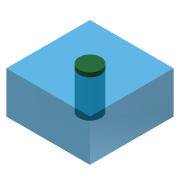
# Autodesk Inventor part: Remnant
Saved by Autodesk Inventor 2014 (Build 180170000, 170)
## iProperties
Created: 2015-06-22
Part Number: Remnant
Material: Generic
Document SubType Name: Modeling
Designer: kulkarni
Density: 1 g/cm^3
Appearance: Default
Author: kulkarni
Autodesk Inventor part; units mm, degrees
ref_plane "YZ Plane" through (0, 0, 0) normal (1, 0, 0) x (0, 1, 0)
ref_plane "XZ Plane" through (0, 0, 0) normal (0, 1, 0) x (-1, 0, 0)
ref_plane "XY Plane" through (0, 0, 0) normal (0, 0, 1) x (1, 0, 0)
sketch "Sketch1" plane through (0, 0, 0) normal (0, 1, 0) x (-1, 0, 0)
  line L0 (0, 0) -> (25.4, 0)
  line L1 (25.4, 0) -> (25.4, -25.4)
  line L2 (25.4, -25.4) -> (0, -25.4)
  line L3 (0, -25.4) -> (0, 0)
  dimension "d0" = 25.4
  dimension "d1" = 25.4
  constraints: 8 end point, 2 parallel, 1 horizontal, 1 perpendicular
  measures "d0" distance of L1.end L2.end
  measures "d1" distance of L0.end L1.end
extrude "Extrusion1" add sketch "Sketch1" along normal blind 12.7
sketch "Sketch2" plane through (0, 12.7, 0) normal (0, 1, 0) x (1, 0, 0)
  circle A0 centre (-12.7, 12.7) radius 3.3294
  constraints: 1 centre point
extrude "Extrusion2" add sketch "Sketch2" along normal blind 1.27 and the other way blind 11.43 separate body
body "Solid1"
body "Solid2"
